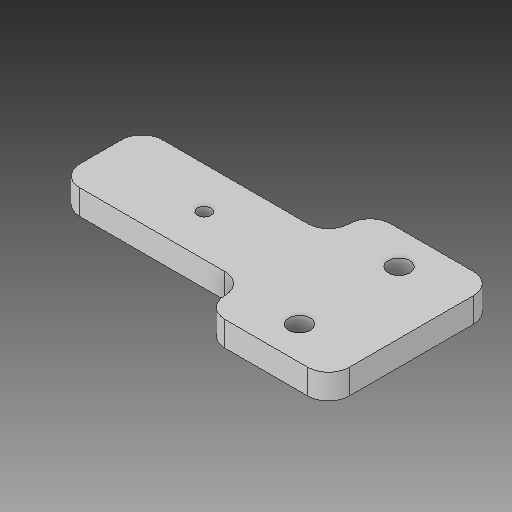
# Autodesk Inventor part: LCD-Plate
Saved by Autodesk Inventor 2018 (Build 220112000, 112)
## iProperties
Created: 2016-07-27
Part Number: LCD-Plate
Material: Generic
Document SubType Name: Modeling
Designer: User
Density: 1 g/cm^3
Appearance: Default
Author: User
Autodesk Inventor part; units mm, degrees
ref_plane "YZ Plane" through (0, 0, 0) normal (1, 0, 0) x (0, 1, 0)
ref_plane "XZ Plane" through (0, 0, 0) normal (0, 1, 0) x (-1, 0, 0)
ref_plane "XY Plane" through (0, 0, 0) normal (0, 0, 1) x (1, 0, 0)
sketch "Sketch1" plane through (0, 0, 0) normal (0, 1, 0) x (-1, 0, 0)
  line L0 (32.7591, 186.1581) -> (67.7591, 186.1581)
  arc A0 (72.7591, 181.1581) -> (67.7591, 186.1581) centre (67.7591, 181.1581) ccw
  line L1 (72.7591, 181.1581) -> (72.7591, 171.1581)
  arc A1 (67.7591, 166.1581) -> (72.7591, 171.1581) centre (67.7591, 171.1581) ccw
  line L2 (67.7591, 166.1581) -> (32.7591, 166.1581)
  arc A2 (32.7591, 166.1581) -> (27.7591, 161.1581) centre (32.7591, 161.1581) ccw
  arc A3 (22.7591, 156.1581) -> (27.7591, 161.1581) centre (22.7591, 161.1581) ccw
  line L3 (22.7591, 156.1581) -> (2.7591, 156.1581)
  arc A4 (-2.2409, 161.1581) -> (2.7591, 156.1581) centre (2.7591, 161.1581) ccw
  line L4 (-2.2409, 161.1581) -> (-2.2409, 191.1581)
  arc A5 (2.7591, 196.1581) -> (-2.2409, 191.1581) centre (2.7591, 191.1581) ccw
  line L5 (2.7591, 196.1581) -> (22.7591, 196.1581)
  arc A6 (27.7591, 191.1581) -> (22.7591, 196.1581) centre (22.7591, 191.1581) ccw
  arc A7 (27.7591, 191.1581) -> (32.7591, 186.1581) centre (32.7591, 191.1581) ccw
  circle A8 centre (12.7591, 188.1581) radius 2.6
  circle A9 centre (12.7591, 164.1581) radius 2.6
  circle A10 centre (47.7591, 176.1581) radius 1.6
  point P0 (0, 0)
  constraints: 17 tangent, 16 point on circle, 12 end point, 11 centre point, 8 equal radius, 3 parallel, 2 perpendicular
extrude "Extrusion1" add sketch "Sketch1" along normal blind 6
body "Solid1"
